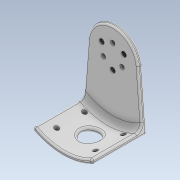
# Autodesk Inventor part: thigh_hip_connector
Saved by Autodesk Inventor 2020 (Build 240168000, 168)
## iProperties
Created: 2021-01-06
Part Number: thigh_hip_connector
Material: Generic
Document SubType Name: Modeling
Designer: DELL
Density: 1 g/cm^3
Appearance: Clear - Blue
Author: DELL
Autodesk Inventor part; units mm, degrees
ref_plane "YZ Plane" through (0, 0, 0) normal (1, 0, 0) x (0, 1, 0)
ref_plane "XZ Plane" through (0, 0, 0) normal (0, 1, 0) x (-1, 0, 0)
ref_plane "XY Plane" through (0, 0, 0) normal (0, 0, 1) x (1, 0, 0)
sketch "Sketch1" plane through (0, 0, 0) normal (0, 0, 1) x (1, 0, 0)
  circle A0 centre (0, 0) radius 22.5
  line L0 (-22.429, 1.7862) -> (-26.5, -49.3331)
  line L1 (22.429, 1.7862) -> (26.5, -49.3331)
  line L2 (9.9593, -5.75) -> (0, 0) construction
  circle A1 centre (8.4134, -4.8575) radius 2
  line L3 (0, 0) -> (9.9593, 5.75) construction
  line L4 (0, 0) -> (-9.9593, -5.75) construction
  circle A2 centre (-8.4134, -4.8575) radius 2
  circle A3 centre (0, 0) radius 9.715 construction
  circle A4 centre (0, 0) radius 11.5 construction
  circle A5 centre (0, 9.715) radius 2
  line L5 (0, 0) -> (-9.9593, 5.75) construction
  line L6 (11.5, 0) -> (-11.5, 0) construction
  circle A6 centre (-9.9593, 5.75) radius 3.75
  circle A7 centre (-9.9593, 5.75) radius 2.25
  line L7 (0, -48.5721) -> (0, 22.5) construction
  circle A8 centre (0, -11.5) radius 2.25
  circle A9 centre (0, -11.5) radius 3.75
  circle A10 centre (9.9593, 5.75) radius 3.75
  circle A11 centre (9.9593, 5.75) radius 2.25
  arc A12 (-26.1506, -44.946) -> (26.1506, -44.946) centre (0, 0) ccw
  arc A13 (-26.5, -49.3331) -> (26.5, -49.3331) centre (0, 0) ccw
  point P0 (0, 11.4686)
  point P1 (0, 11.4686)
  point P2 (11.5, 0)
  point P3 (-11.5, 0)
  dimension "d18" = 23
  dimension "d0" = 45
  dimension "d17" = 19.43
  dimension "d19" = 30
  dimension "d20" = 30
  dimension "d21" = 4.5
  dimension "d22" = 7.5
  dimension "d23" = 4
  dimension "d24" = 104
  dimension "d25" = 112
  dimension "d48" = 53
  constraints: 14 end point, 13 centre point, 10 coincident, 9 point on circle, 8 point on line, 6 equal radius, 2 tangent, 1 vertical, 17 other
  measures "d0" diameter of A0
  measures "d17" diameter of A3
  measures "d19" angle to the sketch x axis of L5
  measures "d20" angle to the sketch x axis of L4
  measures "d21" diameter of A11
  measures "d22" diameter of A10
  measures "d23" diameter of A5
  measures "d24" diameter of A12
  measures "d25" diameter of A13
  measures "d48" distance of L1.end L0.end
extrude "Extrusion1" add sketch "Sketch1" along normal blind 4 contours A0 | A0 L1 A12 L0 | L1 A13 L0 A12 | A1 | A2 | A5 | A6 | A9 | A10
extrude "Extrusion2" cut sketch "Sketch1" along normal blind 3.5 contours A6 | A9 | A10 | A11
extrude "Extrusion3" cut sketch "Sketch1" against normal blind 5 from surface at 4 contours A1 | A2 | A5
extrude "Extrusion4" add sketch "Sketch1" along normal blind 45 from surface at 4 contours L1 A13 L0 A12
fillet "Fillet1" radius 5 1 edges at (0, -52, 4)
fillet "Fillet2" radius 1.5 17 edges at (0, -56, 0) (0, -56, 49) (26.5, -49.3331, 24.5) (-26.5, -49.3331, 24.5) (-24.4645, -23.7734, 0) (24.4645, -23.7734, 0) (0, 22.5, 0) (-24.0669, -18.7809, 4) (-26.0116, -43.2008, 5.3595) (-26.1506, -44.946, 29) (24.0669, -18.7809, 4) (26.0116, -43.2008, 5.3595) (26.1506, -44.946, 29) (0, 22.5, 4) (0, -52, 49) (-26.3253, -47.1395, 49) (26.3253, -47.1395, 49)
sketch "Sketch2" plane through (0, 0, 0) normal (0, 1, 0) x (-1, 0, 0)
  line L0 (-26.3353, 0) -> (-26.3353, 49) construction
  line L1 (20.9337, 0) -> (-20.9337, 0) construction
  line L2 (24.84, 49) -> (-24.84, 49) construction
  line L3 (-26.3353, 24.5) -> (26.4215, 24.5) construction
  line L4 (26.4215, 47.5) -> (26.4215, 1.5) construction
  line L5 (-26.3353, 47.5) -> (-26.3353, 9) construction
  line L6 (0, 0) -> (0, 49) construction
  circle A0 centre (0, 24.5) radius 8
  circle A1 centre (0, 24.5) radius 25
  line L7 (-17.5, 37) -> (17.5, 37) construction
  line L8 (17.5, 37) -> (17.5, 12) construction
  line L9 (17.5, 12) -> (-17.5, 12) construction
  line L10 (-17.5, 12) -> (-17.5, 37) construction
  line L11 (-17.5, 37) -> (17.5, 12) construction
  line L12 (17.5, 37) -> (-17.5, 12) construction
  circle A2 centre (17.5, 12) radius 2
  circle A3 centre (17.5, 12) radius 1.25
  circle A4 centre (-17.5, 12) radius 2
  circle A5 centre (-17.5, 12) radius 1.25
  circle A6 centre (17.5, 37) radius 2
  circle A7 centre (17.5, 37) radius 1.25
  circle A8 centre (-17.5, 37) radius 2
  circle A9 centre (-17.5, 37) radius 1.25
  dimension "d40" = 16
  dimension "d41" = 50
  dimension "d50" = 25
  dimension "d51" = 35
  dimension "d52" = 2.5
  dimension "d53" = 4
  constraints: 18 end point, 10 centre point, 6 coincident, 6 midpoint, 6 symmetric about line, 2 parallel, 2 point on line, 1 collinear, 1 horizontal, 1 perpendicular, 1 vertical, 6 other
  measures "d40" diameter of A0
  measures "d41" diameter of A1
  measures "d50" distance of L7.end L8.end
  measures "d51" distance of L8.end L9.end
  measures "d52" diameter of A3
  measures "d53" diameter of A2
extrude "Extrusion5" cut sketch "Sketch2" against normal through all contours A0 | A3 | A5 | A7 | A9
extrude "Extrusion6" cut sketch "Sketch2" against normal blind 51 contours A2 | A3 | A4 | A5 | A6 | A7 | A8 | A9
fillet "Fillet3" radius 2 2 edges at (8, -51.3809, 24.4769) (8, -55.4256, 24.4768)
body "Solid1"
